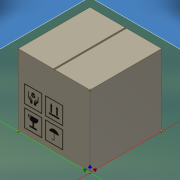
# Autodesk Inventor part: Box - Package
Saved by Autodesk Inventor 2015 (Build 190159000, 159)
## iProperties
Category: Package
Company: IMAGINiT Technologies
Created: 2012-01-09
Part Number: Box - Package
Material: Generic
Document SubType Name: Modeling
Designer: Rusty
Density: 1 g/cm^3
Description: =Package - <Length> x <Width> x <Height>
Appearance: Light Beige
Width: 12.000 in
Height: 12.000 in
Length: 12.000 in
Key Parameters: Width=12.000 in;Height=12.000 in;Length=12.000 in;
Author: Rusty Belcher
Title: Box - Package
Keywords: Box - Package
Comments: Parameters for Length - Width - Height
Autodesk Inventor part; units mm, degrees
ref_plane "YZ Plane" through (0, 0, 0) normal (1, 0, 0) x (0, 1, 0)
ref_plane "XZ Plane" through (0, 0, 0) normal (0, 1, 0) x (-1, 0, 0)
ref_plane "XY Plane" through (0, 0, 0) normal (0, 0, 1) x (1, 0, 0)
sketch "Sketch1" plane through (0, 0, 0) normal (0, 0, 1) x (1, 0, 0)
  line L0 (-152.4, 304.8) -> (152.4, 304.8)
  line L1 (152.4, 304.8) -> (152.4, 0)
  line L2 (152.4, 0) -> (-152.4, 0)
  line L3 (-152.4, 0) -> (-152.4, 304.8)
  point P0 (0, 0)
  point P1 (0, 0)
  constraints: 8 end point, 2 parallel, 1 coincident, 1 horizontal, 1 horizontal alignment, 1 midpoint, 1 perpendicular, 1 vertical alignment
extrude "Extrusion1" add sketch "Sketch1" along normal mid plane 304.8
sketch "Sketch2" plane through (0, 0, 152.4) normal (0, 0, 1) x (1, 0, 0)
  line L0 (-152.4, 304.8) -> (152.4, 304.8) projected
  line L1 (-3.175, 304.8) -> (3.175, 304.8)
  line L2 (3.175, 304.8) -> (3.175, 301.625)
  line L3 (3.175, 301.625) -> (-3.175, 301.625)
  line L4 (-3.175, 301.625) -> (-3.175, 304.8)
  point P0 (0, 0)
  point P1 (0, 304.8)
  dimension "d4" = 3.175
  dimension "d5" = 6.35
  constraints: 8 end point, 2 midpoint, 2 parallel, 1 horizontal, 1 perpendicular, 1 point on line
  measures "d4" distance of L3.end L1.start
  measures "d5" distance of L2.end L3.end
extrude "Extrusion2" cut sketch "Sketch2" against normal through all
sketch "Sketch3" plane through (0, 0, 152.4) normal (0, 0, 1) x (1, 0, 0)
  line L0 (-152.4, 0) -> (-152.4, 304.8) projected
  line L1 (152.4, 0) -> (-152.4, 0) projected
  line L2 (-127, 25.4) -> (-50.8, 25.4)
  line L3 (-50.8, 25.4) -> (-50.8, 101.6)
  line L4 (-50.8, 101.6) -> (-127, 101.6)
  line L5 (-127, 101.6) -> (-127, 25.4)
  line L6 (-123.825, 98.425) -> (-53.975, 98.425)
  line L7 (-53.975, 98.425) -> (-53.975, 28.575)
  line L8 (-53.975, 28.575) -> (-123.825, 28.575)
  line L9 (-123.825, 28.575) -> (-123.825, 98.425)
  line L10 (-38.1, 25.4) -> (38.1, 25.4)
  line L11 (38.1, 25.4) -> (38.1, 101.6)
  line L12 (38.1, 101.6) -> (-38.1, 101.6)
  line L13 (-38.1, 101.6) -> (-38.1, 25.4)
  line L14 (-34.925, 98.425) -> (34.925, 98.425)
  line L15 (34.925, 98.425) -> (34.925, 28.575)
  line L16 (34.925, 28.575) -> (-34.925, 28.575)
  line L17 (-34.925, 28.575) -> (-34.925, 98.425)
  line L18 (-127, 114.3) -> (-50.8, 114.3)
  line L19 (-50.8, 114.3) -> (-50.8, 190.5)
  line L20 (-50.8, 190.5) -> (-127, 190.5)
  line L21 (-127, 190.5) -> (-127, 114.3)
  line L22 (-123.825, 187.325) -> (-53.975, 187.325)
  line L23 (-53.975, 187.325) -> (-53.975, 117.475)
  line L24 (-53.975, 117.475) -> (-123.825, 117.475)
  line L25 (-123.825, 117.475) -> (-123.825, 187.325)
  line L26 (-38.1, 114.3) -> (38.1, 114.3)
  line L27 (38.1, 114.3) -> (38.1, 190.5)
  line L28 (38.1, 190.5) -> (-38.1, 190.5)
  line L29 (-38.1, 190.5) -> (-38.1, 114.3)
  line L30 (-34.925, 187.325) -> (34.925, 187.325)
  line L31 (34.925, 187.325) -> (34.925, 117.475)
  line L32 (34.925, 117.475) -> (-34.925, 117.475)
  line L33 (-34.925, 117.475) -> (-34.925, 187.325)
  point P0 (0, 0)
  dimension "d8" = 76.2
  dimension "d9" = 25.4
  dimension "d10" = 25.4
  dimension "d11" = 3.175
  dimension "d14" = 88.9
  dimension "d17" = 88.9
  constraints: 64 end point, 4 parallel, 3 perpendicular, 2 collinear, 2 horizontal, 1 vertical, 49 other
  measures "d8" distance of L2.end L3.end
  measures "d9" distance between parallel lines of L0 L5
  measures "d10" distance between parallel lines of L1 L2
  measures "d11" distance between parallel lines of L4 L6
  measures "d14" distance of L3.end L12.start
  measures "d17" distance of L3.end L20.start
split_face "Split1"
split_face "Split2"
split_face "Split3"
split_face "Split4"
split_face "Split5"
split_face "Split6"
split_face "Split7"
split_face "Split8"
sketch "Sketch4" plane through (-123.825, 98.425, 152.4) normal (0, 0, 1) x (1, 0, 0)
  line L0 (0, 0) -> (69.85, 0) projected
  line L1 (0, -69.85) -> (0, 0) projected
  line L2 (69.85, -69.85) -> (0, -69.85) projected
  line L3 (19.0891, -57.15) -> (50.7609, -57.15)
  line L4 (50.7609, -57.15) -> (50.7609, -50.8)
  line L5 (19.0891, -50.8) -> (19.0891, -57.15)
  line L6 (38.1, -50.8) -> (38.1, -34.697)
  line L7 (31.75, -34.697) -> (31.75, -50.8)
  line L8 (19.6575, -12.7) -> (16.6521, -18.8843)
  line L9 (16.6521, -18.8843) -> (20.9342, -18.8843)
  line L10 (20.9342, -18.8843) -> (17.3368, -26.287)
  line L11 (22.15, -12.7) -> (20.3175, -16.4708)
  line L12 (20.3175, -16.4708) -> (24.6183, -16.4708)
  line L13 (24.6183, -16.4708) -> (18.9446, -28.1459)
  line L14 (12.7, -12.7) -> (19.6575, -12.7)
  line L15 (22.15, -12.7) -> (57.15, -12.7)
  arc A0 (12.7, -12.7) -> (17.3368, -26.287) centre (34.925, -12.7) ccw
  arc A1 (18.9446, -28.1459) -> (31.75, -34.697) centre (34.925, -12.7) ccw
  arc A2 (38.1, -34.697) -> (57.15, -12.7) centre (34.925, -12.7) ccw
  line L16 (50.7609, -50.8) -> (38.1, -50.8)
  line L17 (31.75, -50.8) -> (19.0891, -50.8)
  point P0 (123.825, -98.425)
  point P1 (34.925, -50.8)
  point P2 (34.925, -29.1715)
  point P3 (34.925, 0)
  dimension "d20" = 12.7
  dimension "d21" = 6.35
  dimension "d22" = 6.35
  dimension "d24" = 12.7
  constraints: 30 end point, 10 parallel, 6 point on circle, 3 centre point, 3 perpendicular, 2 vertical alignment, 1 coincident, 1 horizontal, 1 midpoint
  measures "d20" distance between parallel lines of L3 L2
  measures "d21" distance of L3.end L4.end
  measures "d22" distance between parallel lines of L6 L7
  measures "d24" distance from line of L1 L14.start
split_face "Split9"
split_face "Split10"
sketch "Sketch5" plane through (-34.925, 98.425, 152.4) normal (0, 0, 1) x (1, 0, 0)
  line L0 (69.85, 0) -> (69.85, -69.85) projected
  line L1 (0, 0) -> (69.85, 0) projected
  line L2 (0, -69.85) -> (0, 0) projected
  line L3 (69.85, -69.85) -> (0, -69.85) projected
  line L4 (57.15, -12.7) -> (57.15, -57.15) construction
  line L5 (57.15, -57.15) -> (12.7, -57.15) construction
  line L6 (12.7, -57.15) -> (12.7, -12.7) construction
  line L7 (12.7, -12.7) -> (57.15, -12.7) construction
  line L8 (36.0188, -31.0952) -> (36.0188, -51.4628)
  line L9 (33.8312, -51.4628) -> (33.8312, -31.0952)
  arc A0 (24.6443, -51.4628) -> (36.0188, -51.4628) centre (30.3316, -51.4628) ccw
  arc A1 (26.8319, -51.4628) -> (33.8312, -51.4628) centre (30.3316, -51.4628) ccw
  line L10 (24.6443, -51.4628) -> (26.8319, -51.4628)
  line L11 (36.0188, -13.8321) -> (36.0188, -12.7)
  line L12 (36.0188, -12.7) -> (33.8312, -12.7)
  line L13 (33.8312, -12.7) -> (33.8312, -13.8301)
  arc A2 (23.1675, -30.5813) -> (12.7, -30.0146) centre (17.5638, -37.131) ccw
  arc A3 (33.8312, -30.1527) -> (23.1675, -30.5813) centre (28.7712, -37.131) ccw
  arc A4 (46.5876, -30.5012) -> (36.0188, -30.1527) centre (41.0788, -37.131) ccw
  arc A5 (57.15, -30.1481) -> (46.5876, -30.5012) centre (52.0963, -37.131) ccw
  line L14 (36.0188, -31.0952) -> (36.0188, -30.1527)
  line L15 (33.8312, -31.0952) -> (33.8312, -30.1527)
  arc A6 (57.15, -30.1481) -> (36.0188, -13.8321) centre (34.9039, -37.1178) ccw
  arc A7 (33.8312, -13.8301) -> (12.7, -30.0146) centre (34.9039, -37.1178) ccw
  point P0 (34.925, -98.425)
  point P1 (34.925, -31.0952)
  point P2 (34.925, -31.0952)
  point P3 (34.925, -12.7)
  dimension "d25" = 12.7
  constraints: 24 end point, 16 point on circle, 8 centre point, 3 equal radius, 3 horizontal alignment, 3 parallel, 3 tangent, 2 collinear, 2 midpoint, 2 point on line, 1 coincident, 1 concentric, 1 perpendicular, 3 other
  measures "d25" distance between parallel lines of L1 L7
split_face "Split11"
sketch "Sketch6" plane through (-34.925, 187.325, 152.4) normal (0, 0, 1) x (1, 0, 0)
  line L0 (69.85, 0) -> (69.85, -69.85) projected
  line L1 (0, 0) -> (69.85, 0) projected
  line L2 (0, -69.85) -> (0, 0) projected
  line L3 (69.85, -69.85) -> (0, -69.85) projected
  line L4 (57.15, -12.7) -> (57.15, -57.15) construction
  line L5 (57.15, -57.15) -> (12.7, -57.15)
  line L6 (12.7, -57.15) -> (12.7, -12.7) construction
  line L7 (12.7, -12.7) -> (57.15, -12.7) construction
  line L8 (12.7, -50.8) -> (57.15, -50.8)
  line L9 (22.6976, -12.7) -> (17.5193, -23.9944)
  line L10 (27.8758, -23.9944) -> (22.6976, -12.7)
  line L11 (25.8726, -23.9944) -> (25.8726, -48.0363)
  line L12 (25.8726, -48.0363) -> (19.5226, -48.0363)
  line L13 (19.5226, -48.0363) -> (19.5226, -23.9944)
  line L14 (34.925, -12.7) -> (34.925, -7.7199) construction
  line L15 (47.1524, -12.7) -> (52.3307, -23.9944)
  line L16 (41.9742, -23.9944) -> (47.1524, -12.7)
  line L17 (43.9774, -23.9944) -> (43.9774, -48.0363)
  line L18 (43.9774, -48.0363) -> (50.3274, -48.0363)
  line L19 (50.3274, -48.0363) -> (50.3274, -23.9944)
  line L20 (12.7, -50.8) -> (12.7, -57.15)
  line L21 (57.15, -50.8) -> (57.15, -57.15)
  line L22 (17.5193, -23.9944) -> (19.5226, -23.9944)
  line L23 (25.8726, -23.9944) -> (27.8758, -23.9944)
  line L24 (52.3307, -23.9944) -> (50.3274, -23.9944)
  line L25 (43.9774, -23.9944) -> (41.9742, -23.9944)
  point P0 (34.925, -187.325)
  point P1 (22.6976, -23.9944)
  point P2 (47.1524, -23.9944)
  dimension "d26" = 12.7
  dimension "d27" = 6.35
  dimension "d28" = 6.35
  constraints: 44 end point, 8 symmetric about line, 4 parallel, 3 point on line, 2 collinear, 1 midpoint, 1 perpendicular, 1 vertical alignment, 3 other
  measures "d26" distance between parallel lines of L1 L7
  measures "d27" distance between parallel lines of L5 L8
  measures "d28" distance between parallel lines of L11 L13
split_face "Split12"
split_face "Split13"
split_face "Split14"
sketch "Sketch7" plane through (-123.825, 187.325, 152.4) normal (0, 0, 1) x (1, 0, 0)
  line L0 (0, -69.85) -> (69.85, -69.85) projected
  line L1 (12.7, -12.7) -> (57.15, -12.7) construction
  line L2 (57.15, -57.15) -> (12.7, -57.15) construction
  line L3 (22.6688, -57.15) -> (22.6688, -52.8524)
  arc A0 (22.6688, -52.8524) -> (20.3647, -47.1054) centre (14.3497, -52.8524) ccw
  line L4 (20.3647, -47.1054) -> (15.1508, -41.6484)
  arc A1 (12.7, -34.925) -> (15.1508, -41.6484) centre (21.5956, -35.4908) ccw
  line L5 (15.875, -19.6032) -> (15.875, -31.6397)
  line L6 (17.6337, -36.0264) -> (26.3364, -45.1349)
  arc A2 (26.3364, -45.1349) -> (28.0331, -43.5138) centre (27.1847, -44.3243) ccw
  line L7 (28.0331, -43.5138) -> (21.521, -36.698)
  arc A3 (23.8166, -34.5047) -> (21.521, -36.698) centre (22.6688, -35.6013) ccw
  line L8 (23.8166, -34.5047) -> (30.3287, -41.3205)
  arc A4 (31.533, -44.3243) -> (30.3287, -41.3205) centre (27.1847, -44.3243) ccw
  line L9 (31.533, -44.3243) -> (31.533, -57.15)
  line L10 (34.925, -12.7) -> (34.925, -57.15) construction
  arc A5 (15.875, -19.6032) -> (12.7, -19.6032) centre (14.2875, -19.6032) ccw
  arc A6 (15.875, -31.6397) -> (17.6337, -36.0264) centre (22.225, -31.6397) ccw
  line L11 (12.7, -34.925) -> (12.7, -19.6032)
  line L12 (47.1812, -57.15) -> (47.1812, -52.8524)
  arc A7 (49.4853, -47.1054) -> (47.1812, -52.8524) centre (55.5003, -52.8524) ccw
  line L13 (49.4853, -47.1054) -> (54.6992, -41.6484)
  arc A8 (54.6992, -41.6484) -> (57.15, -34.925) centre (48.2544, -35.4908) ccw
  line L14 (53.975, -19.6032) -> (53.975, -31.6397)
  line L15 (52.2163, -36.0264) -> (43.5136, -45.1349)
  arc A9 (41.8169, -43.5138) -> (43.5136, -45.1349) centre (42.6653, -44.3243) ccw
  line L16 (41.8169, -43.5138) -> (48.329, -36.698)
  arc A10 (48.329, -36.698) -> (46.0334, -34.5047) centre (47.1812, -35.6013) ccw
  line L17 (46.0334, -34.5047) -> (39.5213, -41.3205)
  arc A11 (39.5213, -41.3205) -> (38.317, -44.3243) centre (42.6653, -44.3243) ccw
  line L18 (38.317, -44.3243) -> (38.317, -57.15)
  arc A12 (57.15, -19.6032) -> (53.975, -19.6032) centre (55.5625, -19.6032) ccw
  arc A13 (52.2163, -36.0264) -> (53.975, -31.6397) centre (47.625, -31.6397) ccw
  line L19 (38.317, -57.15) -> (47.1812, -57.15)
  line L20 (57.15, -19.6032) -> (57.15, -34.925)
  line L21 (34.925, -12.7) -> (26.384, -18.361)
  line L22 (26.384, -18.361) -> (34.925, -24.0221)
  line L23 (34.925, -24.0221) -> (43.466, -18.361)
  line L24 (43.466, -18.361) -> (34.925, -12.7)
  line L25 (26.5258, -20.3104) -> (33.8787, -25.1839)
  line L26 (33.8787, -25.1839) -> (33.8787, -33.5217)
  line L27 (33.8787, -33.5217) -> (26.5258, -28.6482)
  line L28 (26.5258, -28.6482) -> (26.5258, -20.3104)
  line L29 (43.3242, -20.3104) -> (35.9713, -25.1839)
  line L30 (35.9713, -25.1839) -> (35.9713, -33.5217)
  line L31 (35.9713, -33.5217) -> (43.3242, -28.6482)
  line L32 (43.3242, -28.6482) -> (43.3242, -20.3104)
  line L33 (22.6688, -57.15) -> (31.533, -57.15)
  line L34 (57.15, -12.7) -> (57.15, -34.925) construction
  line L35 (57.15, -36.0566) -> (57.15, -57.15) construction
  line L36 (12.7, -57.15) -> (12.7, -36.0566) construction
  line L37 (12.7, -34.925) -> (12.7, -12.7) construction
  point P0 (123.825, -187.325)
  dimension "d30" = 12.7
  dimension "d32" = 3.175
  dimension "d33" = 6.35
  constraints: 74 end point, 30 point on circle, 27 symmetric about line, 14 centre point, 14 tangent, 12 parallel, 4 point on line, 2 collinear, 2 midpoint, 1 concentric, 1 horizontal alignment, 1 perpendicular, 7 other
  measures "d30" distance between parallel lines of L0 L2
  measures "d32" distance between parallel lines of L8 L7
  measures "d33" radius of A6
split_face "Split15"
split_face "Split16"
split_face "Split17"
split_face "Split18"
split_face "Split19"
sketch "Sketch8" plane through (-152.4, 304.8, -152.4) normal (0, 1, 0) x (1, 0, 0)
  line L0 (149.225, -304.8) -> (149.225, 0) projected
  line L1 (149.225, 0) -> (0, 0) projected
  line L2 (0, 0) -> (0, -304.8) projected
  line L3 (0, -304.8) -> (149.225, -304.8) projected
  line L4 (0, 0) -> (304.8, -304.8)
  point P0 (152.4, -152.4)
  constraints: 2 end point, 1 midpoint
sketch "Sketch9" plane through (0, 0, -152.4) normal (0, 0, -1) x (-1, 0, 0)
  line L0 (-3.175, 301.625) -> (-3.175, 304.8) projected
  line L1 (-152.4, 304.8) -> (-3.175, 304.8) projected
  line L2 (-152.4, 0) -> (-152.4, 304.8) projected
  line L3 (152.4, 0) -> (-152.4, 0) projected
  line L4 (152.4, 304.8) -> (152.4, 0) projected
  line L5 (3.175, 304.8) -> (152.4, 304.8) projected
  line L6 (3.175, 304.8) -> (3.175, 301.625) projected
  line L7 (3.175, 301.625) -> (-3.175, 301.625) projected
  line L8 (152.4, 304.8) -> (-152.4, 0)
  point P0 (0, 0)
  point P1 (0, 152.4)
  constraints: 2 end point, 1 midpoint
sketch "Sketch10" plane through (-152.4, 0, 152.4) normal (0, 0, 1) x (1, 0, 0)
  line L0 (101.6, 25.4) -> (101.6, 101.6) projected
  line L1 (25.4, 25.4) -> (101.6, 25.4) projected
  line L2 (25.4, 101.6) -> (25.4, 25.4) projected
  line L3 (101.6, 101.6) -> (25.4, 101.6) projected
  line L4 (155.575, 304.8) -> (155.575, 301.625) projected
  line L5 (155.575, 301.625) -> (149.225, 301.625) projected
  line L6 (149.225, 301.625) -> (149.225, 304.8) projected
  line L7 (0, 304.8) -> (149.225, 304.8) projected
  line L8 (0, 0) -> (0, 304.8) projected
  line L9 (304.8, 0) -> (0, 0) projected
  line L10 (304.8, 304.8) -> (304.8, 0) projected
  line L11 (155.575, 304.8) -> (304.8, 304.8) projected
  line L12 (101.6, 190.5) -> (101.6, 114.3) projected
  line L13 (101.6, 114.3) -> (25.4, 114.3) projected
  line L14 (25.4, 114.3) -> (25.4, 190.5) projected
  line L15 (25.4, 190.5) -> (101.6, 190.5) projected
  line L16 (190.5, 114.3) -> (190.5, 190.5) projected
  line L17 (114.3, 114.3) -> (190.5, 114.3) projected
  line L18 (114.3, 190.5) -> (114.3, 114.3) projected
  line L19 (190.5, 190.5) -> (114.3, 190.5) projected
  line L20 (190.5, 25.4) -> (190.5, 101.6) projected
  line L21 (114.3, 25.4) -> (190.5, 25.4) projected
  line L22 (114.3, 101.6) -> (114.3, 25.4) projected
  line L23 (190.5, 101.6) -> (114.3, 101.6) projected
  line L24 (0, 304.8) -> (304.8, 0)
  point P0 (152.4, 0)
  point P1 (152.4, 152.4)
  constraints: 2 end point, 1 midpoint
equation "\"d28\" = d27"
equation "\"d32\" = d31"
equation "\"d31\" = 3.175"
body "Solid1"
